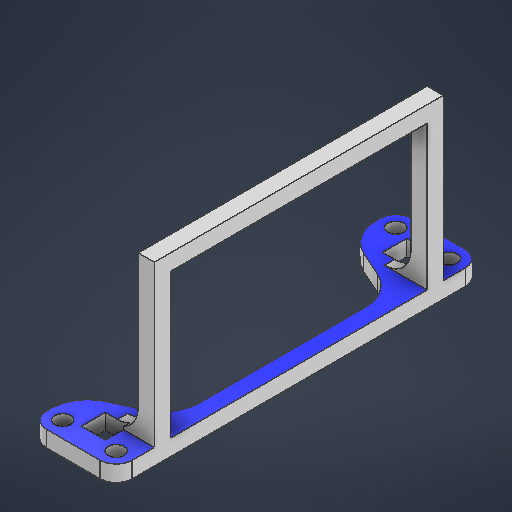
# Autodesk Inventor part: battery_holder_2
Saved by Autodesk Inventor 2026.1 (Build 301233000, 233)
## iProperties
Created: 2026-05-21
Part Number: battery_holder_2
Material: Generic
Document SubType Name: Modeling
Designer: emanuel
Density: 1 g/cm^3
Appearance: Default
Author: emanuel
Autodesk Inventor part; units mm, degrees
ref_plane "YZ Plane" through (0, 0, 0) normal (1, 0, 0) x (0, 1, 0)
ref_plane "XZ Plane" through (0, 0, 0) normal (0, 1, 0) x (-1, 0, 0)
ref_plane "XY Plane" through (0, 0, 0) normal (0, 0, 1) x (1, 0, 0)
sketch "Sketch1" plane through (0, 0, 0) normal (0, 1, 0) x (-1, 0, 0)
  line L0 (-5, 25.15) -> (5, 25.15)
  line L1 (5, 25.15) -> (5, -25.15)
  line L2 (5, -25.15) -> (-5, -25.15)
  line L3 (-5, -25.15) -> (-5, 25.15)
  line L4 (-5, 25.15) -> (5, -25.15) construction
  line L5 (5, 25.15) -> (-5, -25.15) construction
  line L6 (5, 25.15) -> (-5, 25.15)
  line L7 (-5, 25.15) -> (-5, 31.15)
  line L8 (-5, 31.15) -> (5, 31.15)
  line L9 (5, 31.15) -> (5, 25.15)
  line L10 (5, -25.15) -> (-5, -25.15)
  line L11 (-5, -25.15) -> (-5, -31.15)
  line L12 (-5, -31.15) -> (5, -31.15)
  line L13 (5, -31.15) -> (5, -25.15)
  circle A0 centre (5, 31.15) radius 1.5
  circle A1 centre (5, 25.15) radius 1.5
  circle A2 centre (-5, 31.15) radius 1.5
  circle A3 centre (-5, 25.15) radius 1.5
  circle A4 centre (5, -25.15) radius 1.5
  circle A5 centre (5, -31.15) radius 1.5
  circle A6 centre (-5, -25.15) radius 1.5
  circle A7 centre (-5, -31.15) radius 1.5
  line L14 (5, 31.15) -> (8, 31.15)
  line L15 (8, 31.15) -> (8, 34.15)
  line L16 (8, 34.15) -> (5, 34.15)
  line L17 (5, 34.15) -> (5, 31.15)
  line L18 (-5, -31.15) -> (-8, -31.15)
  line L19 (-8, -31.15) -> (-8, -34.15)
  line L20 (-8, -34.15) -> (-5, -34.15)
  line L21 (-5, -34.15) -> (-5, -31.15)
  line L22 (-8, -34.15) -> (8, -34.15)
  line L23 (8, -34.15) -> (8, 34.15)
  line L24 (8, 34.15) -> (-8, 34.15)
  line L25 (-8, 34.15) -> (-8, -34.15)
  line L26 (-2.25, 30.4) -> (2.25, 30.4)
  line L27 (2.25, 30.4) -> (2.25, 25.9)
  line L28 (2.25, 25.9) -> (-2.25, 25.9)
  line L29 (-2.25, 25.9) -> (-2.25, 30.4)
  line L30 (-2.25, 30.4) -> (2.25, 25.9) construction
  line L31 (2.25, 30.4) -> (-2.25, 25.9) construction
  line L32 (-2.25, -25.9) -> (2.25, -25.9)
  line L33 (2.25, -25.9) -> (2.25, -30.4)
  line L34 (2.25, -30.4) -> (-2.25, -30.4)
  line L35 (-2.25, -30.4) -> (-2.25, -25.9)
  line L36 (-2.25, -25.9) -> (2.25, -30.4) construction
  line L37 (2.25, -25.9) -> (-2.25, -30.4) construction
  point P0 (0, 0)
  point P1 (0, 28.15)
  point P2 (0, -28.15)
  dimension "d0" = 10
  dimension "d1" = 50.3
  dimension "d2" = 6
  dimension "d3" = 6
  dimension "d4" = 3
  dimension "d5" = 3
  dimension "d6" = 3
  dimension "d7" = 3
  dimension "d8" = 3
  dimension "d9" = 3
  dimension "d10" = 3
  dimension "d11" = 3
  dimension "d12" = 3
  dimension "d13" = 3
  dimension "d14" = 3
  dimension "d15" = 3
  dimension "d16" = 4.5
  dimension "d17" = 4.5
  dimension "d18" = 4.5
  dimension "d19" = 4.5
  constraints: 76 end point, 16 parallel, 8 centre point, 8 coincident, 8 horizontal, 8 perpendicular, 6 midpoint
  measures "d0" distance of L1.end L2.end
  measures "d1" distance of L0.end L1.end
  measures "d2" distance of L6.end L7.end
  measures "d3" distance of L11.end L10.end
  measures "d4" diameter of A0
  measures "d5" diameter of A1
  measures "d6" diameter of A2
  measures "d7" diameter of A3
  measures "d8" diameter of A4
  measures "d9" diameter of A5
  measures "d10" diameter of A6
  measures "d11" diameter of A7
  measures "d12" distance of L16.end L15.end
  measures "d13" distance of L15.end L14.end
  measures "d14" distance of L20.end L19.end
  measures "d15" distance of L19.end L18.end
  measures "d16" distance of L27.end L28.end
  measures "d17" distance of L26.end L27.end
  measures "d18" distance of L33.end L34.end
  measures "d19" distance of L32.end L33.end
extrude "Extrusion1" add sketch "Sketch1" along normal blind 3 contours L7 A3 L0 | L0 A3 L3 | L3 A3 L7 | A3 L7 A2 L8 A0 L9 A1 L0 | L0 A1 L1 A4 L2 A6 L3 A3 | L3 A6 L11 A7 L18 L25 L24 L17 A0 L8 A2 L7 A3 | A1 L9 L0 | L0 L1 A1 | A6 L2 L3 | L3 L11 A6 | L9 A1 L1 | L9 A0 L14 L23 L22 L21 A7 L12 A5 L13 A4 L1 A1 | L2 A6 L11 | L2 A4 L13 A5 L12 A7 L11 A6 | A4 L13 L1 | L1 L2 A4 | L2 L13 A4 | A0 L17 L16 L15 L14 | A7 L21 L20 L19 L18
sketch "Sketch2" plane through (0, 3, 0) normal (0, 1, 0) x (1, 0, 0)
  line L0 (5, -20) -> (-5, -20)
  line L1 (-5, -20) -> (-5, 20)
  line L2 (-5, 20) -> (5, 20)
  line L3 (5, 20) -> (5, -20)
  line L4 (5, -20) -> (-5, 20) construction
  line L5 (-5, -20) -> (5, 20) construction
  point P0 (0, 0)
  dimension "d22" = 10
  dimension "d23" = 40
  constraints: 12 end point, 2 midpoint, 2 parallel, 1 horizontal, 1 perpendicular
  measures "d22" distance of L1.end L2.end
  measures "d23" distance of L0.end L1.end
extrude "Extrusion2" cut sketch "Sketch2" against normal blind 3
sketch "Sketch3" plane through (0, 3, 0) normal (0, 1, 0) x (1, 0, 0)
  line L0 (8, -34.15) -> (8, 34.15) projected
  line L1 (-8, 24) -> (8, 24)
  line L2 (8, 24) -> (8, -24)
  line L3 (8, -24) -> (-8, -24)
  line L4 (-8, -24) -> (-8, 24)
  line L5 (-8, 24) -> (8, -24) construction
  line L6 (8, 24) -> (-8, -24) construction
  line L7 (8, 24) -> (5, 24)
  line L8 (5, 24) -> (5, 27)
  line L9 (5, 27) -> (8, 27)
  line L10 (8, 27) -> (8, 24)
  line L11 (8, -24) -> (5, -24)
  line L12 (5, -24) -> (5, -27)
  line L13 (5, -27) -> (8, -27)
  line L14 (8, -27) -> (8, -24)
  point P0 (0, 0)
  point P1 (8, 27)
  point P2 (8, -27)
  dimension "d26" = 48
  dimension "d27" = 3
  dimension "d28" = 3
  dimension "d29" = 3
  dimension "d30" = 3
  constraints: 28 end point, 6 parallel, 3 horizontal, 3 perpendicular, 2 midpoint, 1 point on line
  measures "d26" distance of L1.end L2.end
  measures "d27" distance of L8.end L9.end
  measures "d28" distance of L7.end L8.end
  measures "d29" distance of L13.end L12.end
  measures "d30" distance of L12.end L11.end
extrude "Extrusion3" add sketch "Sketch3" along normal blind 27 contours L13 L12 L3 L0 | L1 L8 L9 L0
sketch "Sketch4" plane through (0, 30, 0) normal (0, 1, 0) x (1, 0, 0)
  line L0 (5, 27) -> (8, 27) projected
  line L1 (8, -34.15) -> (8, -27) projected
  line L2 (5, 27) -> (8, 27)
  line L3 (8, 27) -> (8, -27)
  line L4 (8, -27) -> (5, -27)
  line L5 (5, -27) -> (5, 27)
  point P0 (0, 0)
  point P1 (8, 27)
  constraints: 8 end point, 2 parallel, 1 horizontal, 1 perpendicular
extrude "Extrusion4" add sketch "Sketch4" along normal blind 3
sketch "Sketch5" plane through (0, 3, 0) normal (0, 1, 0) x (1, 0, 0)
  line L0 (-2.25, -25.9) -> (2.25, -25.9) projected
  line L1 (-8, 34.15) -> (-8, -34.15) projected
  line L2 (-2.25, -25.9) -> (-8, -25.9)
  line L3 (-8, -25.9) -> (-8, 25.9)
  line L4 (-8, 25.9) -> (-2.25, 25.9)
  line L5 (-2.25, 25.9) -> (-2.25, -25.9)
  line L6 (5, 20) -> (5, -20) projected
  line L7 (5, 20) -> (-8, 25.9)
  line L8 (5, -20) -> (-5, -20) projected
  line L9 (5, -20) -> (-8, -25.9)
  point P0 (0, 0)
  dimension "d35" = 51.8
  constraints: 12 end point, 2 parallel, 1 horizontal, 1 perpendicular, 1 point on line
  measures "d35" distance of L2.end L3.end
extrude "Extrusion5" cut sketch "Sketch5" against normal blind 3 contours L7 L5 L9 L1 | L7 L6 L8 L5 | L5 L8 L9
fillet "Fillet1" radius 7 4 edges at (5, 1.5, 20) (-8, 1.5, 25.9) (-8, 1.5, -25.9) (5, 1.5, -20)
fillet "Fillet2" radius 5 2 edges at (5, 3, -25.5) (5, 3, 25.5)
fillet "Fillet3" radius 3 4 edges at (-8, 1.5, 34.15) (8, 1.5, 34.15) (-8, 1.5, -34.15) (8, 1.5, -34.15)
body "Solid1"
